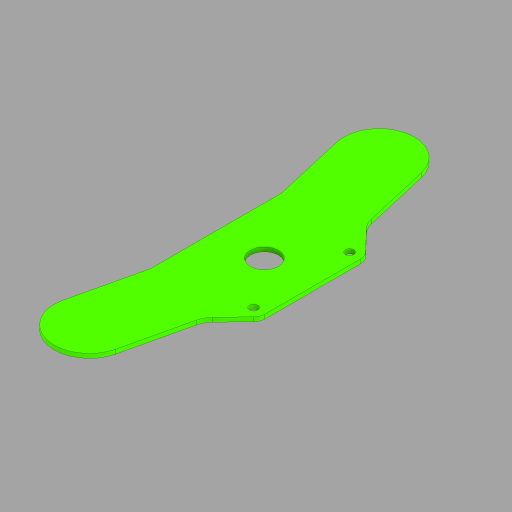
# Autodesk Inventor part: Capasitor_board
Saved by Autodesk Inventor 2024.2 (Build 282272000, 272)
## iProperties
Created: 2024-01-20
Part Number: Capasitor_board
Material: Типовые
Document SubType Name: Modeling
Designer: Fedor Orlov
Density: 1 g/cm^3
Appearance: По умолчанию
Author: Fedor Orlov
Autodesk Inventor part; units mm, degrees
ref_plane "YZ Plane" through (0, 0, 0) normal (1, 0, 0) x (0, 1, 0)
ref_plane "XZ Plane" through (0, 0, 0) normal (0, 1, 0) x (-1, 0, 0)
ref_plane "XY Plane" through (0, 0, 0) normal (0, 0, 1) x (1, 0, 0)
sketch "Эскиз2" plane through (0, 0, 0) normal (0, 1, 0) x (-1, 0, 0)
  line L0 (0, 26) -> (0, -26) construction
  arc A0 (-12.5, 26) -> (-12.1796, 28.8119) centre (0, 26) ccw construction
  line L1 (0, 26) -> (5.8487, 51.3336) construction
  arc A1 (18.0284, 48.5217) -> (-6.3309, 54.1455) centre (5.8487, 51.3336) ccw
  line L2 (0, 0) -> (59.5469, 0) construction
  line L3 (18.0284, 48.5217) -> (12.1796, 23.1881)
  line L4 (-6.3309, 54.1455) -> (-11.682, 30.9675)
  arc A2 (3.0368, 39.154) -> (18.0284, 48.5217) centre (5.8487, 51.3336) ccw construction
  arc A3 (-6.3309, 54.1455) -> (3.0368, 39.154) centre (5.8487, 51.3336) ccw construction
  arc A4 (-12.1796, -28.8119) -> (-12.5, -26) centre (0, -26) ccw construction
  arc A5 (-6.3309, -54.1455) -> (18.0284, -48.5217) centre (5.8487, -51.3336) ccw
  line L5 (18.0284, -48.5217) -> (12.1796, -23.1881)
  line L6 (-6.3309, -54.1455) -> (-11.682, -30.9675)
  arc A6 (18.0284, -48.5217) -> (3.0368, -39.154) centre (5.8487, -51.3336) ccw construction
  arc A7 (3.0368, -39.154) -> (-6.3309, -54.1455) centre (5.8487, -51.3336) ccw construction
  line L7 (12.1796, 23.1881) -> (12.1796, -23.1881)
  arc A8 (-12.1796, 28.8119) -> (-12.5, 26) centre (0, 26) ccw construction
  arc A9 (-12.5, -26) -> (-12.1796, -28.8119) centre (0, -26) ccw construction
  line L8 (-18, 17) -> (-18, -17) construction
  circle A10 centre (-18, 17) radius 1.5
  circle A11 centre (-18, -17) radius 1.5
  arc A12 (-20.8814, 19.7744) -> (-22, 17) centre (-18, 17) ccw
  arc A13 (-18, -13) -> (-22, -17) centre (-18, -17) ccw construction
  line L9 (-22, 17) -> (-22, -17)
  line L10 (-20.8814, 19.7744) -> (-13.7141, 27.2183)
  arc A14 (-13.7141, 27.2183) -> (-11.682, 30.9675) centre (-19.4769, 32.7671) ccw
  arc A15 (-18, 13) -> (-20.8814, 19.7744) centre (-18, 17) ccw construction
  arc A16 (-22, 17) -> (-18, 13) centre (-18, 17) ccw construction
  arc A17 (-22, -17) -> (-20.8814, -19.7744) centre (-18, -17) ccw
  line L11 (-13.7141, -27.2183) -> (-20.8814, -19.7744)
  arc A18 (-11.682, -30.9675) -> (-13.7141, -27.2183) centre (-19.4769, -32.7671) ccw
  arc A19 (-20.8814, -19.7744) -> (-18, -13) centre (-18, -17) ccw construction
  circle A20 centre (-4.794, 0) radius 5
  point P0 (-18, 0)
  point P1 (0, 0)
  dimension "d14" = 52
  dimension "d15" = 26
  dimension "d16" = 25
  dimension "d17" = 26
  dimension "d18" = 167
  dimension "d19" = 25
  dimension "d20" = 34
  dimension "d21" = 18
  dimension "d22" = 3
  dimension "d23" = 3
  dimension "d24" = 8
  dimension "d25" = 8
  dimension "d26" = 8
  dimension "d27" = 8
  dimension "d28" = 10
  dimension "d29" = 4.794
  dimension "d32" = 26
  dimension "d33" = 51.3336
  dimension "d34" = 4.794
  dimension "d35" = 10.6427
  constraints: 38 point on circle, 24 end point, 21 centre point, 17 tangent, 9 point on line, 7 symmetric about line, 6 coincident, 3 midpoint, 3 vertical, 1 horizontal, 4 other
  measures "d14" distance of L0.start L0.end
  measures "d15" distance of L2.start L0.start
  measures "d16" diameter of A0
  measures "d17" distance of L1.start L1.end
  measures "d18" angle of L0 L1
  measures "d19" diameter of A1
  measures "d20" distance of L8.start L8.end
  measures "d21" distance from line of point (0, 0) L8
  measures "d22" diameter of A10
  measures "d23" diameter of A11
  measures "d24" diameter of A12
  measures "d25" diameter of A13
  measures "d26" radius of A14
  measures "d27" radius of A18
  measures "d28" diameter of A20
  measures "d29" distance from line of A20.centre L0
  measures "d32" vertical distance of L0.start A20.centre
  measures "d33" vertical distance of A20.centre L1.end
  measures "d34" horizontal distance of A20.centre L0.start
  measures "d35" horizontal distance of L1.end A20.centre
extrude "Выдавливание2" add sketch "Эскиз2" along normal blind 1.5
